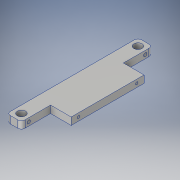
# Autodesk Inventor part: Slide rod connector
Saved by Autodesk Inventor 2017 (Build 210142000, 142)
## iProperties
Created: 2016-12-06
Part Number: Slide rod connector
Material: Aluminum 6061
Document SubType Name: Modeling
Designer: qupec
Density: 2.7 g/cm^3
Appearance: Aluminum - Flat
Mass: 17.588 g
Surface Area: 36.1401 cm^2
Volume: 6.51407 cm^3
Author: qupec
Autodesk Inventor part; units mm, degrees
ref_plane "YZ Plane" through (0, 0, 0) normal (1, 0, 0) x (0, 1, 0)
ref_plane "XZ Plane" through (0, 0, 0) normal (0, 1, 0) x (-1, 0, 0)
ref_plane "XY Plane" through (0, 0, 0) normal (0, 0, 1) x (1, 0, 0)
sketch "Sketch1" plane through (0, 0, 0) normal (0, 1, 0) x (-1, 0, 0)
  line L0 (6.35, 57.15) -> (-6.35, 57.15)
  line L1 (-6.35, 57.15) -> (-6.35, -57.15)
  line L2 (-6.35, -57.15) -> (6.35, -57.15)
  line L3 (6.35, -57.15) -> (6.35, 57.15)
  circle A0 centre (0, 50.8) radius 3.556
  circle A1 centre (0, -50.8) radius 3.556
  point P0 (0, 0)
  dimension "d0" = 12.7
  dimension "d2" = 57.15
  dimension "d3" = 114.3
  dimension "d4" = 101.6
  dimension "d5" = 50.8
  dimension "d25" = 7.112
  dimension "d26" = 7.112
  constraints: 8 end point, 2 centre point, 2 parallel, 1 horizontal, 1 perpendicular
  measures "d0" distance of L0.start L0.end
  measures "d2" distance from line of point (0, 0) L0
  measures "d3" distance of L2.end L0.start
  measures "d4" distance of A0.centre A1.centre
  measures "d5" distance of point (0, 0) A1.centre
  measures "d25" diameter of A1
  measures "d26" diameter of A0
extrude "Extrusion1" add sketch "Sketch1" along normal blind 6.35
sketch "Sketch2" plane through (0, 0, 0) normal (0, -1, 0) x (1, 0, 0)
  circle A0 centre (0, -50.8) radius 3.556 projected
  circle A1 centre (0, 50.8) radius 3.556 projected
  point P0 (0, 0)
extrude "Extrusion2" [suppressed]
sketch "Sketch4" plane through (0, 6.35, 0) normal (0, 1, 0) x (1, 0, 0)
  circle A0 centre (-19.05, 15.1999) radius 3
  line L0 (-20.7085, 12.7) -> (-17.3915, 12.7)
  line L1 (-31.75, 12.7) -> (-6.35, 12.7) projected
  line L2 (-6.35, 57.15) -> (-6.35, -57.15) projected
  arc A1 (-16.521, 12.7) -> (-21.579, 12.7) centre (-19.05, 15.1999) ccw
  line L3 (-31.75, 12.7) -> (-6.35, 12.7) projected
  line L4 (-21.579, 12.7) -> (-20.7085, 12.7)
  line L5 (-17.3915, 12.7) -> (-16.521, 12.7)
  point P0 (0, 0)
  dimension "d18" = 6
  dimension "d19" = 3.317
  dimension "d20" = 0
  dimension "d21" = 12.7
  dimension "d22" = 7.112
  constraints: 6 end point, 4 point on circle, 2 centre point, 2 point on line, 1 coincident, 1 horizontal
  measures "d18" diameter of A0
  measures "d19" distance of L0.start L0.end
  measures "d20" distance between parallel lines of L1 L0
  measures "d21" distance from line of L2 A0.centre
  measures "d22" diameter of A1
extrude "Extrusion4" [suppressed]
mirror "Mirror1" [suppressed]
sketch "Sketch6" plane through (0, 0, 0) normal (0, -1, 0) x (1, 0, 0)
  line L0 (-6.35, 57.15) -> (6.35, 57.15) projected
  line L1 (6.35, 57.15) -> (12.7, 57.15)
  line L2 (12.7, 57.15) -> (12.7, -57.15)
  line L3 (12.7, -57.15) -> (6.35, -57.15)
  line L4 (6.35, -57.15) -> (6.35, 57.15)
  line L5 (6.35, -57.15) -> (-6.35, -57.15) projected
  point P0 (0, 0)
  dimension "d44" = 114.3
  dimension "d45" = 114.3
  dimension "d48" = 6.35
  constraints: 8 end point, 2 parallel, 1 horizontal, 1 perpendicular
  measures "d44" distance between parallel lines of L5 L0
  measures "d45" distance between parallel lines of L3 L1
  measures "d48" distance of L0.end L1.end
extrude "Extrusion6" [suppressed]
ref_plane "Work Plane2" through (12.7, 0, 41.275) normal (1, 0, 0) x (0, 0, -1)
ref_plane "Work Plane3" through (14.2875, 0, 41.275) normal (1, 0, 0) x (0, 0, -1)
ref_plane "Work Plane1" through (12.7, 0, 41.275) normal (1, 0, 0) x (0, 0, -1)
ref_plane "Work Plane4" through (12.7, 3.175, 41.275) normal (0, 1, 0) x (1, 0, 0)
sketch "Sketch11" plane through (0, 6.35, 0) normal (0, 1, 0) x (1, 0, 0)
  circle A0 centre (0, 50.8) radius 3.556 projected
  line L0 (6.35, 57.15) -> (-6.35, 57.15) projected
  circle A1 centre (0, -48.895) radius 3.556 projected
  point P0 (0, 0)
  dimension "d70" = 6.35
  dimension "d71" = 7.112
  dimension "d72" = 97.79
  measures "d70" distance from line of A0.centre L0
  measures "d71" diameter of A0
sketch "Sketch12" plane through (0, 0, 0) normal (0, -1, 0) x (1, 0, 0)
  circle A0 centre (0, 50.8) radius 3.556 projected
  circle A1 centre (0, -50.8) radius 3.556 projected
  circle A2 centre (0, -50.8) radius 1.651
  circle A3 centre (0, 50.8) radius 1.651
  point P0 (0, 0)
  dimension "d73" = 3.302
  dimension "d74" = 3.302
  constraints: 2 centre point, 2 coincident
  measures "d73" diameter of A2
  measures "d74" diameter of A3
extrude "Extrusion11" [suppressed]
sketch "Sketch14" plane through (6.35, 0, 57.15) normal (1, 0, 0) x (0, 0, -1)
  circle A0 centre (6.35, 3.175) radius 1.4224
  line L0 (2.794, 6.35) -> (9.906, 6.35) projected
  line L1 (104.394, 6.35) -> (111.506, 6.35) projected
  line L2 (0, 0) -> (114.3, 0) projected
  point P0 (57.15, 0)
  point P1 (2.159, 1.27)
  point P2 (9.271, 1.27)
  point P3 (99.949, 1.27)
  point P4 (107.061, 1.27)
  dimension "d87" = 2.8448
  dimension "d99" = 3.175
  dimension "d100" = 6.35
  dimension "d101" = 7.112
  dimension "d102" = 3.556
  constraints: 1 centre point
  measures "d87" diameter of A0
  measures "d99" distance from line of L0 A0.centre
  measures "d100" distance between parallel lines of L0 L2
  measures "d101" distance of L0.start L0.end
  measures "d102" horizontal distance of L0.end A0.centre
extrude "Extrusion13" cut sketch "Sketch14" against normal up to next
thread "Thread3" size "5-40 UNC" class "2B" standard "ANSI Unified Screw Threads" full length
mirror "Mirror3" about plane through (0, 0, 0) normal (0, 0, 1) of "Extrusion13"
thread "Thread4" size "5-40 UNC" class "2B" standard "ANSI Unified Screw Threads" full length
fillet "Fillet1" radius 3.175 4 edges at (6.35, 3.175, 57.15) (-6.35, 3.175, 57.15) (6.35, 3.175, -57.15) (-6.35, 3.175, -57.15)
sketch "Sketch15" plane through (0, 6.35, 0) normal (0, 1, 0) x (1, 0, 0)
  line L0 (6.35, -53.975) -> (6.35, 53.975) projected
  line L1 (6.35, -31.75) -> (24.3434, -31.75)
  line L2 (24.3434, -31.75) -> (24.3434, 31.75)
  line L3 (24.3434, 31.75) -> (6.35, 31.75)
  line L4 (6.35, 31.75) -> (6.35, -31.75)
  point P0 (0, 0)
  dimension "d103" = 63.5
  dimension "d104" = 31.75
  dimension "d105" = 17.9934
  constraints: 8 end point, 2 parallel, 1 horizontal, 1 perpendicular, 1 point on line
  measures "d103" distance between parallel lines of L3 L1
  measures "d104" distance from line of point (0, 0) L1
  measures "d105" distance between parallel lines of L0 L2
extrude "Extrusion14" add sketch "Sketch15" against normal up to surface (6.35 mm away)
sketch "Sketch16" plane through (24.3434, 6.35, 31.75) normal (1, 0, 0) x (0, 0, -1)
  line L0 (0, 0) -> (0, -6.35) projected
  line L1 (0, -6.35) -> (63.5, -6.35) projected
  line L2 (63.5, 0) -> (63.5, -6.35) projected
  line L3 (0, 0) -> (63.5, 0) projected
  line L4 (0, 0) -> (0, -6.35) projected
  line L5 (31.75, 0) -> (31.75, -6.35) construction
  line L6 (85.725, -6.35) -> (-22.225, -6.35) projected
  point P0 (31.75, -6.35)
  point P1 (6.35, -3.175)
  point P2 (57.15, -3.175)
  dimension "d129" = 63.5
  dimension "d130" = 31.75
  dimension "d131" = 25.4
  constraints: 2 end point, 2 midpoint, 1 perpendicular, 1 symmetric about line
  measures "d129" distance between parallel lines of L2 L0
  measures "d130" distance between parallel lines of L5 L0
  measures "d131" distance from line of L5 point (6.35, -3.175)
hole "Hole2" at (24.3434, 3.175, 25.4) at (24.3434, 3.175, -25.4) direction (-1, 0, 0) diameter 2.159 depth 12.7
equation "\"d2\" = 0.5 * d3"
equation "\"d5\" = 0.5 * d4"
equation "\"d26\" = d25"
equation "\"d45\" = d44"
equation "\"d74\" = d73"
equation "\"d99\" = 0.5 * d100"
equation "\"d102\" = 0.5 * d101"
equation "\"d104\" = 0.5 * d103"
equation "\"d130\" = 0.5 * d129"
body "Solid1"
